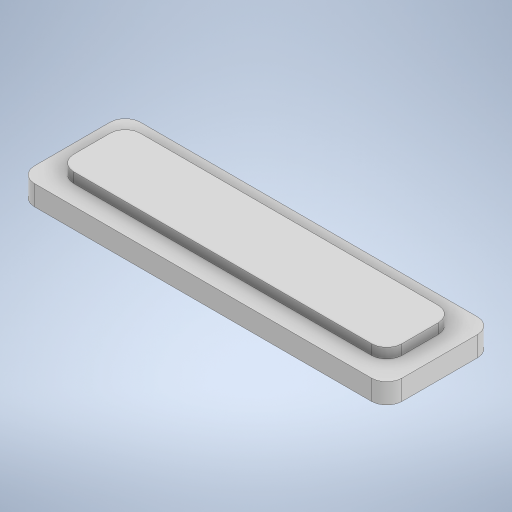
# Autodesk Inventor part: screen3
Saved by Autodesk Inventor 2024 (Build 280153000, 153)
## iProperties
Created: 2023-11-09
Part Number: screen3
Material: Типовые
Document SubType Name: Modeling
Designer: fm
Density: 1 g/cm^3
Appearance: По умолчанию
Author: fm
Autodesk Inventor part; units mm, degrees
ref_plane "YZ Plane" through (0, 0, 0) normal (1, 0, 0) x (0, 1, 0)
ref_plane "XZ Plane" through (0, 0, 0) normal (0, 1, 0) x (-1, 0, 0)
ref_plane "XY Plane" through (0, 0, 0) normal (0, 0, 1) x (1, 0, 0)
sketch "Эскиз1" plane through (0, 0, 0) normal (0, 1, 0) x (-1, 0, 0)
  line L0 (-3.45, 1.95) -> (-32.95, 1.95)
  line L1 (-34.45, 3.45) -> (-34.45, 7.05)
  line L2 (-32.95, 8.55) -> (-3.45, 8.55)
  line L3 (-1.95, 7.05) -> (-1.95, 3.45)
  line L4 (-1.5, 0) -> (-34.9, 0)
  line L5 (-36.4, 1.5) -> (-36.4, 9)
  line L6 (-34.9, 10.5) -> (-1.5, 10.5)
  line L7 (0, 9) -> (0, 1.5)
  arc A0 (-3.45, 1.95) -> (-1.95, 3.45) centre (-3.45, 3.45) ccw
  arc A1 (-1.95, 7.05) -> (-3.45, 8.55) centre (-3.45, 7.05) ccw
  arc A2 (-32.95, 8.55) -> (-34.45, 7.05) centre (-32.95, 7.05) ccw
  arc A3 (-34.45, 3.45) -> (-32.95, 1.95) centre (-32.95, 3.45) ccw
  arc A4 (-36.4, 1.5) -> (-34.9, 0) centre (-34.9, 1.5) ccw
  arc A5 (-34.9, 10.5) -> (-36.4, 9) centre (-34.9, 9) ccw
  arc A6 (0, 9) -> (-1.5, 10.5) centre (-1.5, 9) ccw
  arc A7 (-1.5, 0) -> (0, 1.5) centre (-1.5, 1.5) ccw
  point P0 (0, 0)
  point P1 (-34.45, 1.95)
  point P2 (-1.95, 8.55)
  point P3 (0, 0)
  point P4 (-36.4, 10.5)
  dimension "d6" = 1.5
  dimension "d7" = 1.5
  dimension "d8" = 1.5
  dimension "d9" = 1.5
  dimension "d10" = 1.5
  dimension "d11" = 1.5
  dimension "d12" = 1.5
  dimension "d13" = 1.5
  constraints: 16 end point, 16 point on circle, 16 tangent, 8 centre point, 8 point on line, 4 parallel, 2 horizontal, 2 perpendicular, 1 coincident
  measures "d6" radius of A0
  measures "d7" radius of A1
  measures "d8" radius of A2
  measures "d9" radius of A3
  measures "d10" radius of A4
  measures "d11" radius of A5
  measures "d12" radius of A6
  measures "d13" radius of A7
extrude "Выдавливание3" add sketch "Эскиз1" against normal blind 1 contours L0 A3 L1 A2 L2 A1 L3 A0
extrude "Выдавливание4" add sketch "Эскиз1" against normal blind 2 from surface at -1 contours L0 A3 L1 A2 L2 A1 L3 A0 | L4 A4 L5 A5 L6 A6 L7 A7
